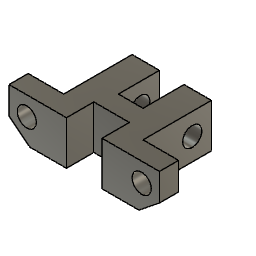
3D Plancha 4 (Autodesk Fusion 360 design; units mm, degrees)
Autodesk Fusion 360 part; units mm, degrees
sketch "Boceto1" plane through (0, 0, 0) normal (0, 0, 1) x (1, 0, 0)
  line L0 (0, 0) -> (4.5, 0)
  line L1 (4.5, 0) -> (4.5, 15)
  line L2 (4.5, 15) -> (14.5, 15)
  line L3 (14.5, 15) -> (14.5, -10)
  line L4 (14.5, -10) -> (27.5, -10)
  line L5 (27.5, -10) -> (27.5, -17)
  line L6 (0, -7) -> (6.5, -7)
  line L7 (6.5, -7) -> (6.5, -17)
  line L8 (6.5, -17) -> (27.5, -17)
  line L9 (0, -7) -> (-6.5, -7)
  line L10 (-27.5, -10) -> (-27.5, -17)
  line L11 (-6.5, -7) -> (-6.5, -17)
  line L12 (-6.5, -17) -> (-27.5, -17)
  line L13 (-14.5, -10) -> (-27.5, -10)
  line L14 (-4.5, 0) -> (-4.5, 15)
  line L15 (-14.5, 15) -> (-14.5, -10)
  line L16 (0, 0) -> (-4.5, 0)
  line L17 (-4.5, 15) -> (-14.5, 15)
  dimension "d1" = 4.5
  dimension "d2" = 15
  dimension "d3" = 10
  dimension "d4" = 25
  dimension "d5" = 13
  dimension "d6" = 7
  dimension "d7" = 6.5
  dimension "d8" = 7
  dimension "d9" = 32
  constraint coincident L0.start L16.start
  constraint horizontal L0
  constraint perpendicular L0 L1
  constraint perpendicular L1 L2
  constraint perpendicular L2 L3
  constraint perpendicular L3 L4
  constraint perpendicular L4 L5
  constraint parallel L0 L6
  constraint perpendicular L0 L7
  measures "d1" distance of L0.start L0.end
  measures "d2" distance of L0.end L1.end
  measures "d3" distance of L1.end L2.end
  measures "d4" distance of L2.end L3.end
  measures "d5" distance of L3.end L4.end
  measures "d6" distance of L4.end L5.end
  measures "d7" distance of L6.start L6.end
  measures "d8" distance of L0.start L6.start
  measures "d9" vertical distance of L2.end L5.end
extrude "Extruir1" add sketch "Boceto1" along normal blind 16
sketch "Boceto2" plane through (0, 0, 0) normal (1, 0, 0) x (0, 1, 0)
  circle A0 centre (8, 8.0871) radius 3.5
  line L0 (15, 0) -> (15, 16)
  dimension "d12" = 7
  dimension "d13" = 7
  measures "d12" diameter of A0
  measures "d13" distance of A0.centre L0
sketch "Boceto3" plane through (-14.5, 0, 0) normal (-1, 0, 0) x (0, -1, 0)
  line L0 (-15, 0) -> (10, 0)
  line L1 (10, 0) -> (10, 16)
  line L2 (10, 16) -> (-15, 16)
  line L3 (-15, 16) -> (-15, 0)
  circle A0 centre (-8, 8) radius 3.5
  dimension "d14" = 7
  measures "d14" diameter of A0
extrude "Extruir2" cut sketch "Boceto2" along normal blind 20
extrude "Extruir3" cut sketch "Boceto3" against normal blind 20 contours A0
sketch "Boceto4" plane through (0, -10, 0) normal (0, 1, 0) x (-1, 0, 0)
  line L0 (-27.5, 0) -> (-14.5, 0)
  line L1 (-14.5, 0) -> (-14.5, 16)
  line L2 (-14.5, 16) -> (-27.5, 16)
  line L3 (-27.5, 16) -> (-27.5, 0)
  line L4 (-27.5, 0) -> (-20, 0)
  line L5 (-27.5, 6) -> (-27.5, 0)
  line L6 (-27.5, 6) -> (-20, 0)
  constraint horizontal L4
  constraint vertical L5
  constraint coincident L0.start L3.end
extrude "Extruir4" cut sketch "Boceto4" against normal blind 8 contours L0 L3 L4 L5 L6
mirror "Simetría1" about plane through (0, 0, 0) normal (1, 0, 0) of "Extruir4"
sketch "Boceto5" plane through (0, -10, 0) normal (0, 1, 0) x (-1, 0, 0)
  line L0 (-27.5, 6) -> (-20, 0)
  line L1 (-20, 0) -> (-14.5, 0)
  line L2 (-14.5, 0) -> (-14.5, 16)
  line L3 (-14.5, 16) -> (-27.5, 16)
  line L4 (-27.5, 16) -> (-27.5, 6)
  circle A0 centre (-21, 9) radius 3.5
  dimension "d27" = 7
  dimension "d28" = 7
  measures "d27" diameter of A0
  measures "d28" distance of L3 A0.centre
extrude "Extruir5" cut sketch "Boceto5" against normal blind 10 contours A0
mirror "Simetría2" about plane through (0, 0, 0) normal (1, 0, 0) of "Extruir5"
